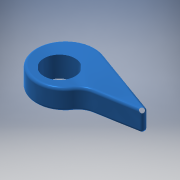
# Autodesk Inventor part: Infill3DExtruderTensionCam
Saved by Autodesk Inventor 2016 (Build 200138000, 138)
## iProperties
Created: 2015-05-04
Part Number: Infill3DExtruderTensionCam
Material: ABS Plastic
Document SubType Name: Modeling
Designer: Jack
Density: 1.06 g/cm^3
Appearance: Cyan
Author: Jack
Autodesk Inventor part; units mm, degrees
ref_plane "YZ Plane" through (0, 0, 0) normal (1, 0, 0) x (0, 1, 0)
ref_plane "XZ Plane" through (0, 0, 0) normal (0, 1, 0) x (-1, 0, 0)
ref_plane "XY Plane" through (0, 0, 0) normal (0, 0, 1) x (1, 0, 0)
sketch "Sketch1" plane through (0, 0, 0) normal (0, 0, 1) x (1, 0, 0)
  arc A0 (3.3974, 9.4052) -> (9.3315, -3.5948) centre (0, 0) ccw
  line L0 (3.3974, 9.4052) -> (29.434, 0)
  line L1 (9.3315, -3.5948) -> (29.434, 0)
  dimension "d0" = 20
  dimension "d33" = 30
  dimension "d34" = 13
  constraints: 4 end point, 2 point on circle, 1 centre point, 1 coincident, 1 horizontal alignment, 1 tangent
  measures "d0" diameter of A0
  measures "d33" angle of L1 L0
  measures "d34" vertical distance of L0.start L1.start
extrude "Extrusion1" add sketch "Sketch1" along normal blind 7
sketch "Sketch2" plane through (0, 0, 7) normal (0, 0, 1) x (1, 0, 0)
  arc A0 (3.3974, 9.4052) -> (9.3315, -3.5948) centre (0, 0) ccw projected
  point P0 (0, -2)
  dimension "d12" = 2
  constraints: 1 vertical alignment
  measures "d12" distance of A0.centre point (0, -2)
hole "Hole1" at (0, -2, 7) direction (0, 0, -1) diameter 10.5 depth 8 tip angle 118
fillet "Fillet1" radius 2 1 edges at (29.434, 0, 3.5)
fillet "Fillet2" radius 6 1 edges at (9.3315, -3.5948, 3.5)
fillet "Fillet3" radius 1 8 edges at (-9.5121, -3.0855, 7) (17.1322, -2.1999, 7) (23.7272, 0.4854, 7) (12.9056, 5.9705, 7) (23.7272, 0.4854, 0) (12.9056, 5.9705, 0) (-9.5121, -3.0855, 0) (17.1322, -2.1999, 0)
body "Solid1"
